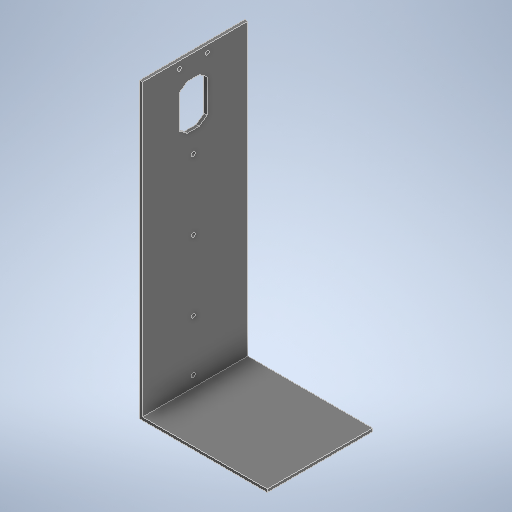
# Autodesk Inventor part: metal Back for v3.1
Saved by Autodesk Inventor 2025 (Build 290162000, 162)
## iProperties
Created: 2025-12-14
Part Number: metal Back for v3.1
Material: Generic
Document SubType Name: Modeling
Designer: kingc
Density: 1 g/cm^3
Appearance: Gray
Author: kingc
Autodesk Inventor part; units mm, degrees
ref_plane "YZ Plane" through (0, 0, 0) normal (1, 0, 0) x (0, 1, 0)
ref_plane "XZ Plane" through (0, 0, 0) normal (0, 1, 0) x (-1, 0, 0)
ref_plane "XY Plane" through (0, 0, 0) normal (0, 0, 1) x (1, 0, 0)
sketch "Sketch1" plane through (0, 0, 0) normal (1, 0, 0) x (0, 1, 0)
  line L0 (114.8402, -25.6502) -> (-118.8398, -25.6502)
  line L1 (-118.8398, -25.6502) -> (-118.8398, -330.4502)
  line L2 (-118.8398, -330.4502) -> (114.8402, -330.4502)
  line L3 (114.8402, -330.4502) -> (114.8402, -25.6502)
  point P0 (0, 0)
  dimension "d0" = 233.68
  dimension "d1" = 304.8
  constraints: 8 end point, 2 parallel, 1 horizontal, 1 perpendicular
  measures "d0" distance of L2.end L1.end
  measures "d1" distance of L1.end L0.end
extrude "Extrusion1" add sketch "Sketch1" along normal blind 2.54
sketch "Sketch2" plane through (2.54, 0, 0) normal (1, 0, 0) x (0, 0, -1)
  line L0 (25.6502, -118.8398) -> (330.4502, -118.8398) projected
  line L1 (25.6502, -118.8398) -> (327.6155, -118.8398)
  line L2 (327.6155, -118.8398) -> (327.6155, -121.3798)
  line L3 (327.6155, -121.3798) -> (25.6502, -121.3798)
  line L4 (25.6502, -121.3798) -> (25.6502, -118.8398)
  point P0 (0, 0)
  dimension "d4" = 2.54
  constraints: 8 end point, 2 parallel, 1 horizontal, 1 perpendicular
  measures "d4" distance of L1.end L2.end
extrude "Extrusion2" add sketch "Sketch2" along normal blind 101.6 and the other way blind 2.54
sketch "Sketch3" plane through (2.54, 0, 0) normal (1, 0, 0) x (0, 0, -1)
  line L0 (115.0337, 99.5367) -> (124.9397, 99.5367)
  line L1 (115.0337, 63.0877) -> (124.9397, 63.0877)
  line L2 (108.7599, 94.9012) -> (108.7599, 67.7232)
  line L3 (131.2135, 67.7232) -> (131.2135, 94.9012)
  line L4 (119.9867, 99.5367) -> (119.9867, 63.0877)
  line L5 (119.9867, 81.3122) -> (117.9124, 81.3122)
  line L6 (108.7599, 94.9012) -> (115.0337, 99.5367)
  line L7 (124.9397, 99.5367) -> (131.2135, 94.9012)
  line L8 (108.7599, 67.7232) -> (115.0337, 63.0877)
  line L9 (124.9397, 63.0877) -> (131.2135, 67.7232)
  line L10 (330.4502, 114.8402) -> (25.6502, 114.8402) projected
  circle A0 centre (108.5567, 111.6652) radius 1.5875
  circle A1 centre (131.4167, 111.6652) radius 1.5875
  circle A2 centre (119.9867, 45.7522) radius 1.5875
  circle A3 centre (119.9867, -11.1438) radius 1.5875
  circle A4 centre (119.9867, -68.0398) radius 1.5875
  circle A5 centre (119.9867, -109.9498) radius 1.5875
  point P0 (0, 0)
  point P1 (108.7599, 81.3122)
  point P2 (119.9867, 63.0877)
  point P3 (131.2135, 81.3122)
  dimension "d9" = 36.449
  dimension "d10" = 22.4536
  dimension "d11" = 11.2268
  dimension "d12" = 9.906
  dimension "d13" = 9.906
  dimension "d14" = 0
  dimension "d15" = 27.178
  dimension "d16" = 27.178
  dimension "d17" = 0
  dimension "d18" = 0
  dimension "d19" = 33.528
  dimension "d20" = 3.175
  dimension "d21" = 3.175
  dimension "d22" = 3.175
  dimension "d23" = 3.175
  dimension "d24" = 11.43
  dimension "d25" = 11.43
  dimension "d26" = 3.175
  dimension "d27" = 3.175
  dimension "d28" = 3.175
  dimension "d29" = 3.175
  dimension "d30" = 0
  dimension "d31" = 0
  dimension "d32" = 0
  dimension "d33" = 69.088
  dimension "d34" = 125.984
  dimension "d35" = 182.88
  dimension "d36" = 224.79
  constraints: 20 end point, 6 centre point, 6 midpoint, 3 horizontal, 2 vertical, 1 perpendicular
  measures "d9" distance from line of L4.start L1
  measures "d10" distance from line of point (108.76, 81.312) L3
  measures "d11" distance between parallel lines of L4 L2
  measures "d12" distance of L0.start L0.end
  measures "d13" distance of L1.start L1.end
  measures "d14" distance from line of L4 point (119.987, 63.088)
  measures "d15" distance of L3.start L3.end
  measures "d16" distance of L2.start L2.end
  measures "d17" vertical distance of L5.start point (131.214, 81.312)
  measures "d18" vertical distance of L5.start point (108.76, 81.312)
  measures "d19" distance from line of L10 L5.start
  measures "d20" diameter of A0
  measures "d21" diameter of A1
  measures "d22" distance from line of L10 A0.centre
  measures "d23" distance from line of L10 A1.centre
  measures "d24" distance from line of L4 A0.centre
  measures "d25" distance from line of A1.centre L4
  measures "d26" diameter of A2
  measures "d27" diameter of A3
  measures "d28" diameter of A4
  measures "d29" diameter of A5
  measures "d30" horizontal distance of A3.centre A2.centre
  measures "d31" horizontal distance of A4.centre A3.centre
  measures "d32" horizontal distance of A5.centre A4.centre
  measures "d33" distance from line of L10 A2.centre
  measures "d34" distance from line of A3.centre L10
  measures "d35" distance from line of L10 A4.centre
  measures "d36" distance from line of L10 A5.centre
extrude "Extrusion3" cut sketch "Sketch3" against normal blind 101.6
sketch "Sketch4" plane through (0, 114.8402, -25.6502) normal (0, 1, 0) x (1, 0, 0)
  line L0 (0, 304.8) -> (0, 0) projected
  line L1 (0, 0) -> (2.54, 0) projected
  line L2 (2.54, 304.8) -> (2.54, 0) projected
  line L3 (0, 304.8) -> (2.54, 304.8) projected
  point P0 (0, -25.6502)
extrude "Extrusion4" add sketch "Sketch4" along normal blind 2.54
sketch "Sketch5" plane through (2.54, -118.8398, -25.6502) normal (0, 1, 0) x (1, 0, 0)
  line L0 (-2.54, 0) -> (0, 0) projected
  line L1 (-2.54, 0) -> (104.5715, 0)
  line L2 (104.5715, 0) -> (104.5715, 52.966)
  line L3 (104.5715, 52.966) -> (-2.54, 52.966)
  line L4 (-2.54, 52.966) -> (-2.54, 0)
  line L5 (101.6, 0) -> (101.6, 301.9653) projected
  line L6 (-2.54, 304.8) -> (101.6, 304.8)
  line L7 (101.6, 304.8) -> (101.6, 138.7986)
  line L8 (101.6, 138.7986) -> (-2.54, 138.7986)
  line L9 (-2.54, 138.7986) -> (-2.54, 304.8)
  point P0 (-2.54, -25.6502)
  point P1 (101.6, 52.966)
  constraints: 16 end point, 4 parallel, 2 horizontal, 2 perpendicular, 2 point on line
extrude "Extrusion5" cut sketch "Sketch5" along normal through all both and the other way through all contours L4 L3 L5 L1 L0 | L8 L9 L6 L7 L5
body "Solid1"
